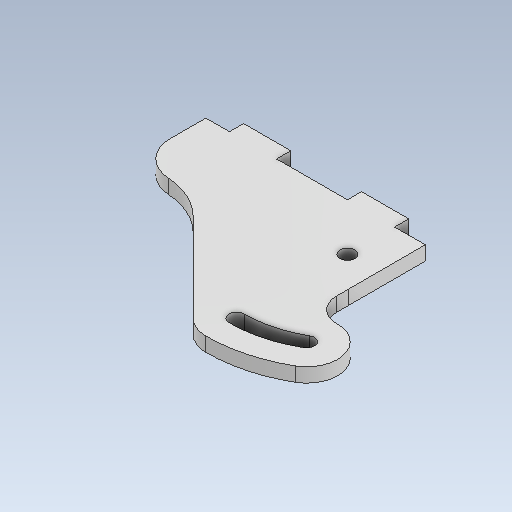
# Autodesk Inventor part: camMount
Saved by Autodesk Inventor 2020 (Build 240168000, 168)
## iProperties
Created: 2019-08-06
Part Number: camMount
Material: Generic
Document SubType Name: Modeling
Designer: n10208577
Density: 1 g/cm^3
Appearance: Default
Author: n10208577
Autodesk Inventor part; units mm, degrees
ref_plane "YZ Plane" through (0, 0, 0) normal (1, 0, 0) x (0, 1, 0)
ref_plane "XZ Plane" through (0, 0, 0) normal (0, 1, 0) x (-1, 0, 0)
ref_plane "XY Plane" through (0, 0, 0) normal (0, 0, 1) x (1, 0, 0)
sketch "Sketch1" plane through (0, 0, 0) normal (0, 1, 0) x (-1, 0, 0)
  arc A0 (14.6882, 29.8139) -> (14.6882, 33.0139) centre (14.6882, 31.4139) ccw
  circle A1 centre (14.6882, 7.9139) radius 1.6
  line L0 (14.6882, -2.0861) -> (8.1882, -2.0861)
  arc A2 (14.6882, 29.8139) -> (3.7382, 26.8799) centre (14.6882, 7.9139) ccw
  arc A3 (14.6882, 33.0139) -> (2.1382, 29.6511) centre (14.6882, 7.9139) ccw
  arc A4 (14.6882, 37.9139) -> (-0.3118, 33.8947) centre (14.6882, 7.9139) ccw
  line L1 (24.6882, -2.0861) -> (24.6882, -5.0861)
  line L2 (24.6882, -5.0861) -> (14.6882, -5.0861)
  line L3 (14.6882, -5.0861) -> (14.6882, -2.0861)
  line L4 (8.1846, 14.2314) -> (8.1882, -2.0861)
  line L5 (39.6882, -2.0861) -> (24.6882, -2.0861)
  line L6 (49.6882, -2.0861) -> (49.6882, -5.0861)
  line L7 (49.6882, -5.0861) -> (39.6882, -5.0861)
  line L8 (39.6882, -5.0861) -> (39.6882, -2.0861)
  line L9 (49.6882, -2.0861) -> (54.6882, -2.0861)
  arc A5 (2.1382, 29.6511) -> (3.7382, 26.8799) centre (2.9382, 28.2655) ccw
  arc A6 (-0.3118, 33.8947) -> (2.9382, 21.7655) centre (2.9382, 28.2655) ccw
  line L10 (8.1846, 14.2314) -> (8.1846, 16.7655)
  arc A7 (8.1846, 16.7655) -> (3.1846, 21.7655) centre (3.1846, 16.7655) ccw
  line L11 (3.1846, 21.7655) -> (2.9382, 21.7655)
  arc A8 (19.2844, 36.0101) -> (14.6882, 37.9139) centre (14.6882, 31.4139) ccw
  line L12 (54.6882, -2.0861) -> (54.6882, 5.4139)
  arc A9 (54.6882, 5.4139) -> (47.6724, 12.8983) centre (47.1882, 5.4139) ccw
  arc A10 (38.0341, 17.2604) -> (47.6724, 12.8983) centre (48.6407, 27.867) ccw
  line L13 (19.2844, 36.0101) -> (38.0341, 17.2604)
  constraints: 28 end point, 20 point on circle, 11 centre point
extrude "Extrusion1" add sketch "Sketch1" along normal blind 3
body "Solid1"
